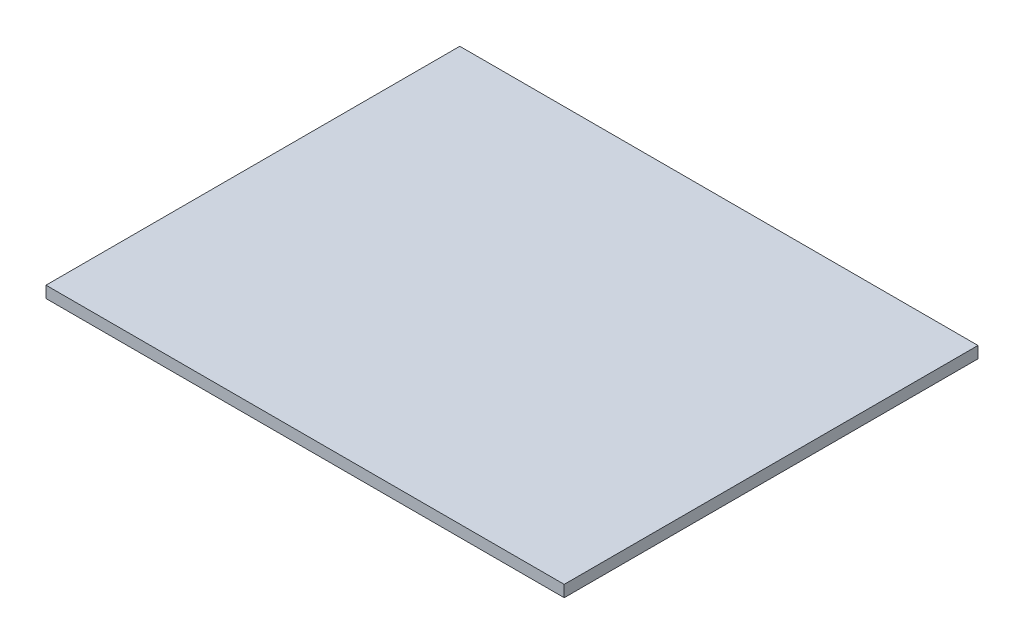
# Autodesk Inventor part: bak
Saved by Autodesk Inventor 2022 (Build 260153000, 153)
## iProperties
Created: 2021-12-16
Part Number: bak
Material: Generic
Document SubType Name: Modeling
Designer: keemi
Density: 1 g/cm^3
Appearance: Default
Author: keemi
Autodesk Inventor part; units mm, degrees
ref_plane "YZ Plane" through (0, 0, 0) normal (1, 0, 0) x (0, 1, 0)
ref_plane "XZ Plane" through (0, 0, 0) normal (0, 1, 0) x (-1, 0, 0)
ref_plane "XY Plane" through (0, 0, 0) normal (0, 0, 1) x (1, 0, 0)
sketch "Sketch1" plane through (0, 0, 0) normal (0, 1, 0) x (-1, 0, 0)
  line L0 (0, 0) -> (-67, 0)
  line L1 (-67, 0) -> (-67, 107)
  line L2 (-67, 107) -> (0, 107)
  line L3 (0, 107) -> (0, 0)
  line L4 (0, 107) -> (67, 107)
  line L5 (67, 107) -> (67, 0)
  line L6 (67, 0) -> (0, 0)
  line L7 (0, 0) -> (0, 107)
  dimension "d0" = 67
  dimension "d1" = 107
  dimension "d2" = 67
  dimension "d3" = 107
  constraints: 16 end point, 4 parallel, 2 horizontal, 2 perpendicular
  measures "d0" distance of L1.end L2.end
  measures "d1" distance of L0.end L1.end
  measures "d2" distance of L5.end L6.end
  measures "d3" distance of L4.end L5.end
extrude "Extrusion1" add sketch "Sketch1" against normal blind 3
body "Solid1"
